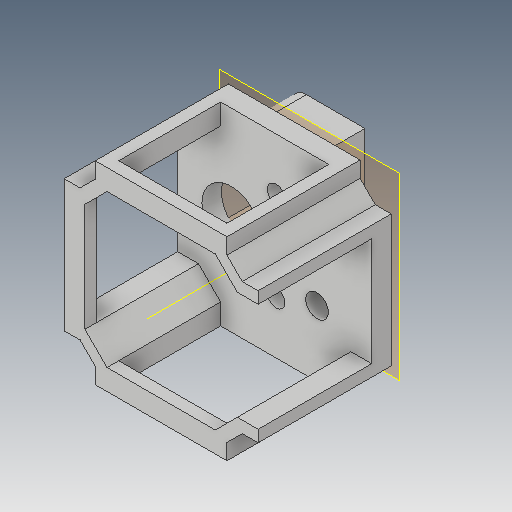
# Autodesk Inventor part: 30_Cube_Z_Focus_Drylin_NEMA_base_v3
Saved by Autodesk Inventor 2019.4 (Build 234330000, 330)
## iProperties
Created: 2021-04-25
Part Number: 30_Cube_Z_Focus_Drylin_NEMA_base_v3
Material: Generic
Document SubType Name: Modeling
Designer: diederichbenedict
Density: 1 g/cm^3
Appearance: Default
Author: diederichbenedict
Autodesk Inventor part; units mm, degrees
ref_plane "Work Plane1" through (0, 0, 0) normal (0, 0, 1) x (1, 0, 0)
sketch "Sketch1" plane through (0, 0, 0) normal (0, 0, 1) x (1, 0, 0)
  arc A0 (12.5934, -5.8404) -> (12.8401, -5.9947) centre (12.8241, -5.7459) ccw construction
  line L0 (12.8401, -5.9947) -> (16.4715, -5.9947) construction
  line L1 (16.4715, -5.9947) -> (16.97, -5.4961) construction
  line L2 (16.97, -5.4961) -> (16.97, 1.583) construction
  arc A1 (16.97, 2.3806) -> (16.97, 1.583) centre (17.2691, 1.9818) ccw construction
  line L3 (16.97, 2.3806) -> (16.97, 5.4715) construction
  line L4 (16.97, 5.4715) -> (16.4715, 5.97) construction
  line L5 (16.4715, 5.97) -> (12.8401, 5.97) construction
  arc A2 (12.8401, 5.97) -> (12.6094, 5.8152) centre (12.8401, 5.7207) ccw construction
  arc A3 (12.0954, 5.2394) -> (12.6094, 5.8152) centre (11.5075, 6.2814) ccw construction
  arc A4 (12.0954, 5.2394) -> (11.974, 5.0466) centre (12.2223, 5.0248) ccw construction
  line L6 (11.974, 5.0466) -> (11.9439, 4.702) construction
  arc A5 (11.6955, 4.4744) -> (11.9439, 4.702) centre (11.6955, 4.7237) ccw construction
  line L7 (11.6955, 4.4744) -> (11.2445, 4.4744) construction
  arc A6 (10.9961, 4.702) -> (11.2445, 4.4744) centre (11.2445, 4.7237) ccw construction
  line L8 (10.9961, 4.702) -> (10.9642, 5.0674) construction
  arc A7 (10.9642, 5.0674) -> (10.8487, 5.2566) centre (10.7158, 5.0457) ccw construction
  arc A8 (10.3792, 5.8152) -> (10.8487, 5.2566) centre (11.4862, 6.2691) ccw construction
  arc A9 (10.3792, 5.8152) -> (10.1485, 5.97) centre (10.1485, 5.7206) ccw construction
  line L9 (10.1485, 5.97) -> (9.4685, 5.97) construction
  line L10 (9.4685, 5.97) -> (8.97, 5.4715) construction
  line L11 (8.97, 5.4715) -> (8.97, -5.4961) construction
  line L12 (8.97, -5.4961) -> (9.4685, -5.9947) construction
  line L13 (9.4685, -5.9947) -> (10.1412, -5.9947) construction
  arc A10 (10.1412, -5.9947) -> (10.3791, -5.84) centre (10.1485, -5.7455) ccw construction
  arc A11 (10.8487, -5.2813) -> (10.3791, -5.84) centre (11.4862, -6.2938) ccw construction
  arc A12 (10.8487, -5.2813) -> (10.9642, -5.0921) centre (10.7158, -5.0704) ccw construction
  line L14 (10.9642, -5.0921) -> (10.9961, -4.7266) construction
  arc A13 (11.2445, -4.4991) -> (10.9961, -4.7266) centre (11.2445, -4.7483) ccw construction
  line L15 (11.2445, -4.4991) -> (11.6955, -4.4991) construction
  arc A14 (11.9439, -4.7266) -> (11.6955, -4.4991) centre (11.6955, -4.7483) ccw construction
  line L16 (11.9439, -4.7266) -> (11.974, -5.0712) construction
  arc A15 (11.974, -5.0712) -> (12.0954, -5.264) centre (12.2223, -5.0495) ccw construction
  arc A16 (12.5934, -5.8404) -> (12.0954, -5.264) centre (11.4862, -6.2938) ccw construction
  arc A17 (24.85, 22.85) -> (22.85, 24.85) centre (22.85, 22.85) ccw construction
  line L17 (22.85, 24.85) -> (-16.97, 24.85) construction
  line L18 (-16.97, 24.85) -> (-16.97, 21.15) construction
  line L19 (-16.97, 21.15) -> (16.97, 21.15) construction
  line L20 (16.97, 16.97) -> (16.97, 21.15) construction
  line L21 (21.15, 16.97) -> (16.97, 16.97) construction
  line L22 (21.15, 16.97) -> (21.15, -16.97) construction
  line L23 (21.15, -16.97) -> (24.85, -16.97) construction
  line L24 (24.85, -16.97) -> (24.85, 22.85) construction
  line L25 (23.75, 23.25) -> (23.75, 18.15) construction
  arc A18 (23.25, 17.65) -> (23.75, 18.15) centre (23.25, 18.15) ccw construction
  line L26 (23.25, 17.65) -> (20.8937, 17.65) construction
  arc A19 (20.5239, 17.8134) -> (20.8937, 17.65) centre (20.8937, 18.15) ccw construction
  line L27 (20.5239, 17.8134) -> (17.7803, 20.8273) construction
  arc A20 (17.65, 21.1639) -> (17.7803, 20.8273) centre (18.15, 21.1639) ccw construction
  line L28 (17.65, 21.1639) -> (17.65, 23.25) construction
  arc A21 (18.15, 23.75) -> (17.65, 23.25) centre (18.15, 23.25) ccw construction
  line L29 (18.15, 23.75) -> (23.25, 23.75) construction
  arc A22 (23.75, 23.25) -> (23.25, 23.75) centre (23.25, 23.25) ccw construction
  arc A23 (-24.85, -22.85) -> (-22.85, -24.85) centre (-22.85, -22.85) ccw construction
  line L30 (-22.85, -24.85) -> (16.97, -24.85) construction
  line L31 (16.97, -24.85) -> (16.97, -21.15) construction
  line L32 (16.97, -21.15) -> (-16.97, -21.15) construction
  line L33 (-16.97, -16.97) -> (-16.97, -21.15) construction
  line L34 (-21.15, -16.97) -> (-16.97, -16.97) construction
  line L35 (-21.15, -16.97) -> (-21.15, 16.97) construction
  line L36 (-21.15, 16.97) -> (-24.85, 16.97) construction
  line L37 (-24.85, 16.97) -> (-24.85, -22.85) construction
  line L38 (-20.8273, -17.7803) -> (-17.8134, -20.5239) construction
  arc A24 (-17.65, -20.8937) -> (-17.8134, -20.5239) centre (-18.15, -20.8937) ccw construction
  line L39 (-17.65, -20.8937) -> (-17.65, -23.25) construction
  arc A25 (-18.15, -23.75) -> (-17.65, -23.25) centre (-18.15, -23.25) ccw construction
  line L40 (-18.15, -23.75) -> (-23.25, -23.75) construction
  arc A26 (-23.75, -23.25) -> (-23.25, -23.75) centre (-23.25, -23.25) ccw construction
  line L41 (-23.75, -23.25) -> (-23.75, -18.15) construction
  arc A27 (-23.25, -17.65) -> (-23.75, -18.15) centre (-23.25, -18.15) ccw construction
  line L42 (-23.25, -17.65) -> (-21.1639, -17.65) construction
  arc A28 (-20.8273, -17.7803) -> (-21.1639, -17.65) centre (-21.1639, -18.15) ccw construction
  arc A29 (-22.85, 24.85) -> (-24.85, 22.85) centre (-22.85, 22.85) ccw construction
  line L43 (-22.85, 24.85) -> (16.97, 24.85) construction
  line L44 (16.97, 24.85) -> (16.97, 21.15) construction
  line L45 (16.97, 21.15) -> (-16.97, 21.15) construction
  line L46 (-16.97, 16.97) -> (-16.97, 21.15) construction
  line L47 (-21.15, 16.97) -> (-16.97, 16.97) construction
  line L48 (-21.15, 16.97) -> (-21.15, -16.97) construction
  line L49 (-21.15, -16.97) -> (-24.85, -16.97) construction
  line L50 (-24.85, -16.97) -> (-24.85, 22.85) construction
  line L51 (-20.8273, 17.7803) -> (-17.8134, 20.5239) construction
  arc A30 (-17.8134, 20.5239) -> (-17.65, 20.8937) centre (-18.15, 20.8937) ccw construction
  line L52 (-17.65, 20.8937) -> (-17.65, 23.25) construction
  arc A31 (-17.65, 23.25) -> (-18.15, 23.75) centre (-18.15, 23.25) ccw construction
  line L53 (-18.15, 23.75) -> (-23.25, 23.75) construction
  arc A32 (-23.25, 23.75) -> (-23.75, 23.25) centre (-23.25, 23.25) ccw construction
  line L54 (-23.75, 23.25) -> (-23.75, 18.15) construction
  arc A33 (-23.75, 18.15) -> (-23.25, 17.65) centre (-23.25, 18.15) ccw construction
  line L55 (-23.25, 17.65) -> (-21.1639, 17.65) construction
  arc A34 (-21.1639, 17.65) -> (-20.8273, 17.7803) centre (-21.1639, 18.15) ccw construction
  arc A35 (22.85, -24.85) -> (24.85, -22.85) centre (22.85, -22.85) ccw construction
  line L56 (22.85, -24.85) -> (-16.97, -24.85) construction
  line L57 (-16.97, -24.85) -> (-16.97, -21.15) construction
  line L58 (-16.97, -21.15) -> (16.97, -21.15) construction
  line L59 (16.97, -16.97) -> (16.97, -21.15) construction
  line L60 (21.15, -16.97) -> (16.97, -16.97) construction
  line L61 (21.15, -16.97) -> (21.15, 16.97) construction
  line L62 (21.15, 16.97) -> (24.85, 16.97) construction
  line L63 (24.85, 16.97) -> (24.85, -22.85) construction
  line L64 (23.75, -23.25) -> (23.75, -18.15) construction
  arc A36 (23.75, -18.15) -> (23.25, -17.65) centre (23.25, -18.15) ccw construction
  line L65 (23.25, -17.65) -> (20.8937, -17.65) construction
  arc A37 (20.8937, -17.65) -> (20.5239, -17.8134) centre (20.8937, -18.15) ccw construction
  line L66 (20.5239, -17.8134) -> (17.7803, -20.8273) construction
  arc A38 (17.7803, -20.8273) -> (17.65, -21.1639) centre (18.15, -21.1639) ccw construction
  line L67 (17.65, -21.1639) -> (17.65, -23.25) construction
  arc A39 (17.65, -23.25) -> (18.15, -23.75) centre (18.15, -23.25) ccw construction
  line L68 (18.15, -23.75) -> (23.25, -23.75) construction
  arc A40 (23.25, -23.75) -> (23.75, -23.25) centre (23.25, -23.25) ccw construction
  circle A41 centre (0.47, -10.47) radius 1.1 construction
  circle A42 centre (0.47, 12.53) radius 1.025 construction
  line L69 (24.85, 16.87) -> (16.87, 16.87)
  line L70 (16.87, 16.87) -> (16.87, -16.87)
  line L71 (16.87, -16.87) -> (24.85, -16.87)
  line L72 (24.85, -16.87) -> (24.85, 16.87)
  line L73 (-16.87, 24.85) -> (16.87, 24.85)
  line L74 (16.87, 24.85) -> (16.87, 13.87)
  line L75 (16.87, 13.87) -> (-16.87, 13.87)
  line L76 (-16.87, 13.87) -> (-16.87, 24.85)
  line L77 (-16.87, 16.87) -> (-24.85, 16.87)
  line L78 (-24.85, 16.87) -> (-24.85, -16.87)
  line L79 (-24.85, -16.87) -> (-16.87, -16.87)
  line L80 (-16.87, -16.87) -> (-16.87, 16.87)
  line L81 (-16.87, -24.85) -> (16.87, -24.85)
  line L82 (16.87, -24.85) -> (16.87, -13.87)
  line L83 (16.87, -13.87) -> (-16.87, -13.87)
  line L84 (-16.87, -13.87) -> (-16.87, -24.85)
  line L85 (16.87, 13.87) -> (-16.87, 13.87)
  line L86 (-16.87, 13.87) -> (-16.87, -13.87)
  line L87 (-16.87, -13.87) -> (16.87, -13.87)
  line L88 (16.87, -13.87) -> (16.87, 13.87)
  point P0 (0, 0)
extrude "Extrusion1" add sketch "Sketch1" along normal blind 5
chamfer "Chamfer1" distance 3.9 angle 45 4 edges at (16.87, -16.87, 2.5) (-16.87, -16.87, 2.5) (-16.87, 16.87, 2.5) (16.87, 16.87, 2.5)
sketch "Sketch2" plane through (0, 0, 5) normal (0, 0, 1) x (1, 0, 0)
  line L0 (16.87, -24.85) -> (16.87, -20.77) projected
  line L1 (-16.87, -20.77) -> (-16.87, -24.85) projected
  line L2 (-16.87, -24.85) -> (16.87, -24.85) projected
  line L3 (20.77, -16.87) -> (16.87, -20.77) projected
  line L4 (20.77, -16.87) -> (24.85, -16.87) projected
  line L5 (24.85, -16.87) -> (24.85, 16.87) projected
  line L6 (24.85, 16.87) -> (20.77, 16.87) projected
  line L7 (16.87, 20.77) -> (20.77, 16.87) projected
  line L8 (16.87, 20.77) -> (16.87, 24.85) projected
  line L9 (16.87, 24.85) -> (-16.87, 24.85) projected
  line L10 (-16.87, 24.85) -> (-16.87, 20.77) projected
  line L11 (-20.77, 16.87) -> (-16.87, 20.77) projected
  line L12 (-20.77, 16.87) -> (-24.85, 16.87) projected
  line L13 (-24.85, 16.87) -> (-24.85, -16.87) projected
  line L14 (-24.85, -16.87) -> (-20.77, -16.87) projected
  line L15 (-16.87, -20.77) -> (-20.77, -16.87) projected
  line L16 (13.8689, -19.5269) -> (13.8689, -21.8489)
  line L17 (-13.8689, -21.8489) -> (-13.8689, -19.5269)
  line L18 (-13.8689, -19.5269) -> (-19.5269, -13.8689)
  line L19 (-19.5269, -13.8689) -> (-21.8489, -13.8689)
  line L20 (-21.8489, 13.8689) -> (-19.5269, 13.8689)
  line L21 (-19.5269, 13.8689) -> (-13.8689, 19.5269)
  line L22 (-13.8689, 19.5269) -> (-13.8689, 21.8489)
  line L23 (13.8689, 21.8489) -> (13.8689, 19.5269)
  line L24 (13.8689, 19.5269) -> (19.5269, 13.8689)
  line L25 (19.5269, 13.8689) -> (21.8489, 13.8689)
  line L26 (21.8489, -13.8689) -> (19.5269, -13.8689)
  line L27 (19.5269, -13.8689) -> (13.8689, -19.5269)
  line L28 (13.8689, -21.8489) -> (13.8689, -24.85)
  line L29 (16.87, -24.85) -> (-16.87, -24.85) projected
  line L30 (21.8489, -13.8689) -> (24.85, -13.8689)
  line L31 (24.85, -16.87) -> (24.85, 16.87) projected
  line L32 (21.8489, 13.8689) -> (24.85, 13.8689)
  line L33 (13.8689, 21.8489) -> (13.8689, 24.85)
  line L34 (-13.8689, 21.8489) -> (-13.8689, 24.85)
  line L35 (-21.8489, 13.8689) -> (-24.85, 13.8689)
  line L36 (-21.8489, -13.8689) -> (-24.85, -13.8689)
  line L37 (-13.8689, -21.8489) -> (-13.8689, -24.85)
  line L38 (13.8689, -21.8489) -> (11.5469, -21.8489)
  line L39 (-11.5469, -21.8489) -> (-13.8689, -21.8489)
  line L40 (21.8489, 13.8689) -> (21.8489, 11.5469)
  line L41 (21.8489, -11.5469) -> (21.8489, -13.8689)
  line L42 (-21.8489, -13.8689) -> (-21.8489, -11.5469)
  line L43 (-21.8489, 11.5469) -> (-21.8489, 13.8689)
  line L44 (-13.8689, 21.8489) -> (-11.5469, 21.8489)
  line L45 (11.5469, 21.8489) -> (13.8689, 21.8489)
  point P0 (0, 0)
  constraints: 56 end point, 20 point on line, 3 perpendicular, 1 parallel, 7 other
ref_plane "Work Plane2" through (-16.97, -24.85, 34.1) normal (0, 0, -1) x (0, 1, 0)
extrude "Extrusion2" add sketch "Sketch2" along normal up to surface (29.1 mm away) contours L2 L28 L16 L27 L26 L30 L5 L4 L3 L0
pattern_circular "Circular Pattern1" count 4 over 360 about axis through (0, 0, 17.13) along (0, 0, -1) of "Extrusion2"
sketch "Sketch3" plane through (-24.85, -13.8689, 34.1) normal (0, 0, 1) x (1, 0, 0)
  circle A0 centre (13.82, 13.8689) radius 1.5 projected
  line L0 (10.9811, -5.658) -> (5.3231, 0) projected
  line L1 (5.3231, 0) -> (0, 0) projected
  line L2 (0, 0) -> (0, -3.0011) projected
  line L3 (0, -3.0011) -> (4.08, -3.0011) projected
  line L4 (4.08, -3.0011) -> (7.98, -6.9011) projected
  line L5 (7.98, -6.9011) -> (7.98, -10.9811) projected
  line L6 (7.98, -10.9811) -> (10.9811, -10.9811) projected
  line L7 (10.9811, -10.9811) -> (10.9811, -5.658) projected
  line L8 (5.3231, 27.7378) -> (10.9811, 33.3958) projected
  line L9 (10.9811, 33.3958) -> (10.9811, 38.7189) projected
  line L10 (10.9811, 38.7189) -> (7.98, 38.7189) projected
  line L11 (7.98, 38.7189) -> (7.98, 34.6389) projected
  line L12 (7.98, 34.6389) -> (4.08, 30.7389) projected
  line L13 (4.08, 30.7389) -> (0, 30.7389) projected
  line L14 (0, 30.7389) -> (0, 27.7378) projected
  line L15 (0, 27.7378) -> (5.3231, 27.7378) projected
  line L16 (10.9811, -10.9811) -> (16.9811, -10.9811)
  line L17 (16.9811, 38.7189) -> (10.9811, 38.7189)
  line L18 (0, 0) -> (0, 27.7378)
  line L19 (0, 0) -> (5.3231, 0)
  line L20 (5.3231, 0) -> (5.3231, 27.7378)
  line L21 (5.3231, 27.7378) -> (0, 27.7378)
  line L22 (0, 27.7378) -> (0, 0)
  line L23 (5.3231, 0) -> (0, 0) projected
  line L24 (5.3231, 0) -> (10.9811, -5.658)
  line L25 (10.9811, 33.3958) -> (5.3231, 27.7378)
  line L26 (38.7189, 38.7189) -> (38.7189, 33.3958) projected
  line L27 (38.7189, -5.658) -> (38.7189, -10.9811) projected
  line L28 (10.9811, -10.9811) -> (38.7189, -10.9811)
  line L29 (38.7189, -10.9811) -> (38.7189, -5.658)
  line L30 (38.7189, -5.658) -> (10.9811, -5.658)
  line L31 (10.9811, -5.658) -> (10.9811, -10.9811)
  line L32 (10.9811, 38.7189) -> (10.9811, 33.3958) projected
  line L33 (10.9811, 38.7189) -> (38.7189, 38.7189)
  line L34 (38.7189, 38.7189) -> (38.7189, 33.3958)
  line L35 (38.7189, 33.3958) -> (10.9811, 33.3958)
  line L36 (10.9811, 33.3958) -> (10.9811, 38.7189)
  line L37 (16.9811, -10.9811) -> (16.9811, -5.658)
  line L38 (16.9811, 33.3958) -> (16.9811, 38.7189)
  line L39 (10.9811, 38.7189) -> (10.9811, 33.3958)
  line L40 (10.9811, -5.658) -> (10.9811, -10.9811)
  line L41 (10.9811, -5.658) -> (10.9811, 0)
  line L42 (10.9811, 27.7378) -> (10.9811, 33.3958)
  line L43 (49.7, 0) -> (44.3769, 0) projected
  line L44 (44.3769, 27.7378) -> (49.7, 27.7378) projected
  line L45 (44.3769, 27.7378) -> (49.7, 27.7378)
  line L46 (49.7, 27.7378) -> (49.7, 0)
  line L47 (49.7, 0) -> (44.3769, 0)
  line L48 (44.3769, 0) -> (44.3769, 27.7378)
  point P0 (24.85, 13.8689)
  dimension "d19" = 6
  constraints: 54 end point, 14 equal length, 6 perpendicular, 5 horizontal, 4 point on line, 3 vertical
  measures "d19" distance of L17.end L17.start
extrude "Extrusion3" add sketch "Sketch3" against normal blind 3 contours L7 L6 L5 L4 L3 L2 L1 L0 | L30 L37 L16 L7 | L1 L18 L15 L20 | L30 L27 L28 L37 | L15 L14 L13 L12 L11 L10 L9 L8 | L9 L17 L38 L35 | L38 L33 L26 L35 | L43 L48 L44 L46
ref_plane "Work Plane3" through (16.97, -5.4961, -37.9) normal (1, 0, 0) x (0, 1, 0)
sketch "Sketch7" plane through (0, 0, 0) normal (0, 0, -1) x (-1, 0, 0)
  arc A0 (18.93, 12.43) -> (22.43, 8.93) centre (22.43, 12.43) ccw construction
  line L0 (18.93, 12.43) -> (18.93, 14.53) construction
  line L1 (3.13, 14.53) -> (18.93, 14.53) construction
  line L2 (3.13, 14.53) -> (3.13, 12.43) construction
  arc A1 (-0.37, 8.93) -> (3.13, 12.43) centre (-0.37, 12.43) ccw construction
  line L3 (-0.37, 8.93) -> (-2.47, 8.93) construction
  line L4 (-2.47, -6.87) -> (-2.47, 8.93) construction
  line L5 (-2.47, -6.87) -> (-0.37, -6.87) construction
  arc A2 (3.13, -10.37) -> (-0.37, -6.87) centre (-0.37, -10.37) ccw construction
  line L6 (3.13, -10.37) -> (3.13, -12.47) construction
  line L7 (18.93, -12.47) -> (3.13, -12.47) construction
  line L8 (18.93, -12.47) -> (18.93, -10.37) construction
  arc A3 (22.43, -6.87) -> (18.93, -10.37) centre (22.43, -10.37) ccw construction
  line L9 (22.43, -6.87) -> (24.53, -6.87) construction
  line L10 (24.53, 8.93) -> (24.53, -6.87) construction
  line L11 (24.53, 8.93) -> (22.43, 8.93) construction
  circle A4 centre (11.03, 1.03) radius 2.5 construction
  arc A5 (-1.5344, 11.2045) -> (0.934, 13.4886) centre (-0.47, 12.53) ccw construction
  circle A6 centre (-0.47, -10.47) radius 1.1 construction
  arc A7 (0.5944, 13.8555) -> (-1.874, 11.5714) centre (-0.47, 12.53) ccw construction
  line L12 (-19.5269, -13.8689) -> (-24.85, -13.8689) construction
  line L13 (-19.5269, 13.8689) -> (-13.8689, 19.5269) construction
  line L14 (-13.8689, 19.5269) -> (-13.8689, 24.85) construction
  line L15 (-13.8689, 24.85) -> (13.8689, 24.85) construction
  line L16 (13.8689, 24.85) -> (13.8689, 19.5269) construction
  line L17 (13.8689, 19.5269) -> (19.5269, 13.8689) construction
  line L18 (19.5269, 13.8689) -> (24.85, 13.8689) construction
  line L19 (24.85, 13.8689) -> (24.85, -13.8689) construction
  line L20 (24.85, -13.8689) -> (19.5269, -13.8689) construction
  line L21 (19.5269, -13.8689) -> (13.8689, -19.5269) construction
  line L22 (13.8689, -19.5269) -> (13.8689, -24.85) construction
  line L23 (13.8689, -24.85) -> (-13.8689, -24.85) construction
  line L24 (-13.8689, -24.85) -> (-13.8689, -19.5269) construction
  line L25 (-13.8689, -19.5269) -> (-19.5269, -13.8689) construction
  line L26 (16.87, 13.87) -> (-16.87, 13.87) construction
  line L27 (16.87, 13.87) -> (-19.5258, 13.87) projected
  line L28 (-2.13, 13.87) -> (16.87, 13.87)
  line L29 (16.87, 13.87) -> (16.87, -16.47)
  line L30 (16.87, -16.47) -> (-2.13, -16.47)
  line L31 (-2.13, -16.47) -> (-2.13, 13.87)
  line L32 (16.97, 16.97) -> (-16.97, 16.97)
  line L33 (16.87, 13.87) -> (-2.13, 13.87)
  line L34 (-2.13, 13.87) -> (-2.13, 16.47)
  line L35 (-2.13, 16.47) -> (16.87, 16.47)
  line L36 (16.87, 16.47) -> (16.87, 13.87)
  line L37 (-16.97, -16.97) -> (16.97, -16.97) construction
  line L38 (-24.85, -13.8689) -> (-24.85, 13.8689) projected
  line L39 (-24.85, 13.8689) -> (-19.5269, 13.8689) projected
  point P0 (0, 0)
  dimension "d35" = 19
  dimension "d54" = 0.5
  dimension "d55" = 0.5
  constraints: 18 end point, 4 parallel, 3 horizontal, 2 perpendicular, 1 point on line, 2 other
  measures "d35" distance between parallel lines of L29 L31
  measures "d54" distance between parallel lines of L35 L32
  measures "d55" distance between parallel lines of L37 L30
ref_plane "Work Plane4" through (-25.03, -12.97, -12) normal (0, 0, 1) x (1, 0, 0)
extrude "Extrusion7" add sketch "Sketch7" along normal blind 16 and the other way blind 5
sketch "Sketch8" plane through (0, 0, 5) normal (0, 0, 1) x (1, 0, 0)
  arc A0 (0.35, -14) -> (2.85, -11.5) centre (0.35, -11.5) ccw projected
  circle A1 centre (0.35, 11.5) radius 1.025 projected
  circle A2 centre (0.35, -11.5) radius 1.025 projected
  point P0 (0, 0)
  point P1 (0.47, 12.53)
  point P2 (0.47, -10.47)
hole "Hole1" at (0.35, 11.5, 5) at (0.35, -11.5, 5) direction (0, 0, -1) diameter 2.5 end through all counterbore diameter 4.5 counterbore depth 16
sketch "Sketch9" plane through (2.13, -16.47, -16) normal (0, 0, -1) x (-1, 0, 0)
  circle A0 centre (13.28, 16.47) radius 13
  point P0 (2.13, 16.47)
  dimension "d93" = 11.15
  constraints: 1 centre point
  measures "d93" distance of point (2.13, 16.47) A0.centre
extrude "Extrusion8" cut sketch "Sketch9" against normal blind 3
sketch "Sketch10" plane through (2.13, -16.47, -13) normal (0, 0, -1) x (-1, 0, 0)
  circle A0 centre (13.28, 16.47) radius 7.5
  arc A1 (19, 28.144) -> (19, 4.796) centre (13.28, 16.47) ccw construction
  point P0 (2.13, 16.47)
  dimension "d49" = 15
  constraints: 1 centre point, 1 coincident
  measures "d49" diameter of A0
extrude "Extrusion9" cut sketch "Sketch10" against normal up to next
fillet "Fillet1" radius 4 2 edges at (-16.87, -16.47, -8) (-16.87, 16.47, -8)
sketch "Sketch14" plane through (0, 0, 5) normal (0, 0, 1) x (1, 0, 0)
  circle A0 centre (-11.15, 0) radius 7.5 projected
  line L0 (13.8689, 19.5269) -> (13.8689, 24.85) projected
  line L1 (13.8689, 24.85) -> (-13.8689, 24.85) projected
  line L2 (-13.8689, 24.85) -> (-13.8689, 19.5269) projected
  line L3 (-13.8689, 19.5269) -> (-19.5269, 13.8689) projected
  line L4 (-19.5269, 13.8689) -> (-24.85, 13.8689) projected
  line L5 (-24.85, 13.8689) -> (-24.85, -13.8689) projected
  line L6 (-24.85, -13.8689) -> (-19.5269, -13.8689) projected
  line L7 (-19.5269, -13.8689) -> (-13.8689, -19.5269) projected
  line L8 (-13.8689, -19.5269) -> (-13.8689, -24.85) projected
  line L9 (-13.8689, -24.85) -> (13.8689, -24.85) projected
  line L10 (13.8689, -24.85) -> (13.8689, -19.5269) projected
  line L11 (13.8689, -19.5269) -> (19.5269, -13.8689) projected
  line L12 (19.5269, -13.8689) -> (24.85, -13.8689) projected
  line L13 (24.85, -13.8689) -> (24.85, 13.8689) projected
  line L14 (24.85, 13.8689) -> (19.5269, 13.8689) projected
  line L15 (19.5269, 13.8689) -> (13.8689, 19.5269) projected
  circle A1 centre (10.85, -8) radius 2.9
  circle A2 centre (10.85, 8) radius 2.9
  point P0 (0, 0)
  dimension "d74" = 5.8
  dimension "d75" = 5.8
  dimension "da" = 8
  dimension "d77" = 8
  dimension "db" = 14
  dimension "d79" = 14
  constraints: 2 centre point
  measures "d74" diameter of A1
  measures "d75" diameter of A2
  measures "da" vertical distance of A2.centre A0.centre
  measures "d77" vertical distance of A0.centre A1.centre
  measures "db" distance from line of L13 A1.centre
  measures "d79" distance from line of L13 A2.centre
extrude "Extrusion12" cut sketch "Sketch14" against normal blind 10 contours A1 | A2
sketch "Sketch17" plane through (-16.87, 24.85, 34.1) normal (0, 0, 1) x (1, 0, 0)
  line L0 (41.72, -10.9811) -> (41.72, -38.7189) projected
  line L1 (36.3969, -38.7189) -> (41.72, -38.7189) projected
  line L2 (36.3969, -38.7189) -> (36.3969, -10.9811) projected
  line L3 (41.72, -10.9811) -> (36.3969, -10.9811) projected
  point P0 (16.87, -24.85)
extrude "Extrusion15" cut sketch "Sketch17" against normal blind 27
equation "\"d77\" = da"
equation "\"d79\" = db"
equation "\"d2\" = d1"
equation "\"d3\" = d1"
equation "\"d4\" = d1"
equation "\"d5\" = d1"
equation "\"d1\" = 0.1"
body "Solid1"
